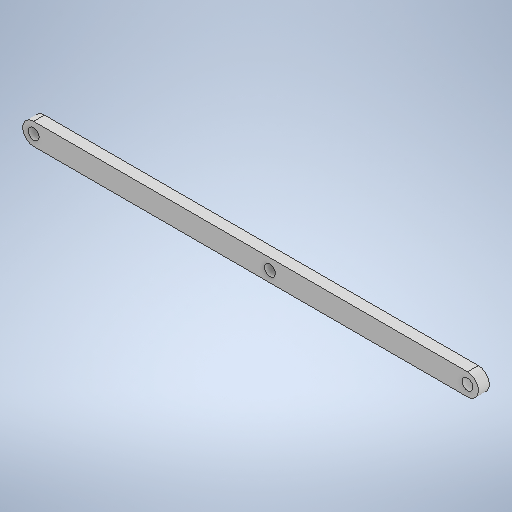
# Autodesk Inventor part: barre_direction
Saved by Autodesk Inventor 2025.1 (Build 291241000, 241)
## iProperties
Created: 2024-10-17
Part Number: barre_direction
Material: Générique
Document SubType Name: Modeling
Designer: baince
Density: 1 g/cm^3
Appearance: Par défaut
Author: baince
Autodesk Inventor part; units mm, degrees
ref_plane "YZ Plane" through (0, 0, 0) normal (1, 0, 0) x (0, 1, 0)
ref_plane "XZ Plane" through (0, 0, 0) normal (0, 1, 0) x (-1, 0, 0)
ref_plane "XY Plane" through (0, 0, 0) normal (0, 0, 1) x (1, 0, 0)
sketch "Esquisse1" plane through (0, 0, 0) normal (0, 0, 1) x (1, 0, 0)
  line L0 (-63, 0) -> (63, 0) construction
  line L1 (-60, -3) -> (60, -3)
  line L2 (60, 3) -> (-60, 3)
  arc A0 (-60, 3) -> (-60, -3) centre (-60, 0) ccw
  arc A1 (60, -3) -> (60, 3) centre (60, 0) ccw
  line L3 (0, -4.2) -> (0, 4.2) projected
  circle A2 centre (-60, 0) radius 1.5
  circle A3 centre (60, 0) radius 1.5
  circle A4 centre (5.35, 0) radius 1.5
  point P0 (0, 0)
  point P1 (0, 0)
  dimension "d0" = 120
  dimension "d1" = 6
  dimension "d2" = 3
  dimension "d4" = 3
  dimension "d7" = 3
  dimension "d9" = 54.65
  constraints: 8 end point, 6 point on circle, 5 centre point, 4 tangent, 3 point on line, 2 coincident, 2 midpoint, 1 horizontal, 1 parallel, 1 symmetric about line
  measures "d0" distance of L2.start L2.end
  measures "d1" distance between parallel lines of L1 L2
  measures "d2" diameter of A2
  measures "d4" diameter of A3
  measures "d7" diameter of A4
  measures "d9" distance of A1.centre A4.centre
extrude "Extrusion1" add sketch "Esquisse1" along normal mid plane 3
